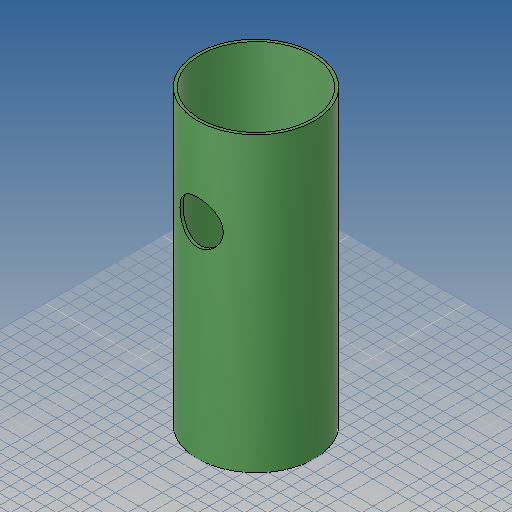
# Autodesk Inventor part: Zyklon_Basis
Saved by Autodesk Inventor 2019 (Build 230136000, 136)
## iProperties
Created: 2020-07-30
Part Number: Zyklon_Basis
Material: Generisch
Document SubType Name: Modeling
Designer: Stefan
Mass: 1480.24 g
Surface Area: 6113.48 cm^2
Volume: 1480.24 cm^3
Density: 1 g/cm^3
Appearance: Glatt - waldgrün
Author: Stefan
Autodesk Inventor part; units mm, degrees
ref_plane "YZ Plane" through (0, 0, 0) normal (1, 0, 0) x (0, 1, 0)
ref_plane "XZ Plane" through (0, 0, 0) normal (0, 1, 0) x (-1, 0, 0)
ref_plane "XY Plane" through (0, 0, 0) normal (0, 0, 1) x (1, 0, 0)
sketch "Skizze1" plane through (0, 0, 0) normal (0, 1, 0) x (-1, 0, 0)
  circle A0 centre (0, 0) radius 100
  circle A1 centre (0, 0) radius 95.1
  dimension "d0" = 200
  dimension "d1" = 4.9
  constraints: 2 centre point, 2 coincident
  measures "d0" diameter of A0
  measures "d1" radial gap between concentric circles of A0 A1
extrude "Extrusion1" add sketch "Skizze1" against normal blind 500
sketch "Skizze2" plane through (0, 0, 0) normal (0, 0, 1) x (1, 0, 0)
  line L0 (0, -224.4) -> (0, 37.4) projected
  circle A0 centre (0, -150) radius 37
  point P0 (0, 0)
  dimension "d4" = 74
  dimension "d6" = 150
  constraints: 1 centre point, 1 point on line
  measures "d4" diameter of A0
  measures "d6" distance of A0.centre point (0, 0)
extrude "Extrusion2" cut sketch "Skizze2" along normal through all
equation "\"d0\" = kg_diameter"
equation "\"d1\" = kg_thickness"
equation "\"kg_diameter\" = 200"
equation "\"kg_thickness\" = 4.9"
equation "\"ht_thickness\" = 1.9"
equation "\"case_thickness\" = 18"
equation "\"gap_slide\" = 0.2"
equation "\"gap_air\" = 1"
equation "\"bore_diameter\" = 73"
equation "\"gap_fit\" = 0.1"
equation "\"mdf_thickness\" = 6"
equation "\"tape_width\" = 15"
equation "\"tape_thickness\" = 3"
equation "\"inner_thickness\" = 15"
equation "\"inner_depth\" = 255"
